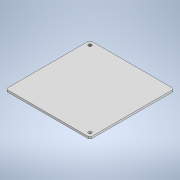
# Autodesk Inventor part: tampa caixa box
Saved by Autodesk Inventor 2022 (Build 260153000, 153)
## iProperties
Created: 2022-04-15
Part Number: tampa caixa box
Material: Genérico
Document SubType Name: Modeling
Designer: Hanter
Density: 1 g/cm^3
Appearance: Padrão
Author: Hanter
Autodesk Inventor part; units mm, degrees
ref_plane "YZ Plane" through (0, 0, 0) normal (1, 0, 0) x (0, 1, 0)
ref_plane "XZ Plane" through (0, 0, 0) normal (0, 1, 0) x (-1, 0, 0)
ref_plane "XY Plane" through (0, 0, 0) normal (0, 0, 1) x (1, 0, 0)
sketch "Esboço1" plane through (0, 0, 0) normal (0, 1, 0) x (-1, 0, 0)
  line L0 (-42.5, 42.5) -> (42.5, 42.5)
  line L1 (42.5, 42.5) -> (42.5, -42.5)
  line L2 (42.5, -42.5) -> (-42.5, -42.5)
  line L3 (-42.5, -42.5) -> (-42.5, 42.5)
  line L4 (-42.5, 42.5) -> (42.5, -42.5) construction
  line L5 (42.5, 42.5) -> (-42.5, -42.5) construction
  point P0 (0, 0)
  dimension "d0" = 85
  dimension "d1" = 85
  constraints: 12 end point, 2 midpoint, 2 parallel, 1 horizontal, 1 perpendicular
  measures "d0" distance of L1.end L2.end
  measures "d1" distance of L0.end L1.end
extrude "Extrusão1" add sketch "Esboço1" along normal blind 2
fillet "Arredondamento1" radius 2 4 edges at (42.5, 1, 42.5) (42.5, 1, -42.5) (-42.5, 1, 42.5) (-42.5, 1, -42.5)
sketch "Esboço2" plane through (0, 2, 0) normal (0, 1, 0) x (1, 0, 0)
  circle A0 centre (38.25, -38.25) radius 1.6
  line L0 (-40.5, -42.5) -> (40.5, -42.5) projected
  line L1 (42.5, -40.5) -> (42.5, 40.5) projected
  circle A1 centre (-38.25, 38.25) radius 1.6
  line L2 (-42.5, 40.5) -> (-42.5, -40.5) projected
  line L3 (40.5, 42.5) -> (-40.5, 42.5) projected
  point P0 (0, 0)
  dimension "d5" = 3.2
  dimension "d6" = 4.25
  dimension "d7" = 4.25
  dimension "d8" = 3.2
  dimension "d9" = 4.25
  dimension "d10" = 4.25
  constraints: 2 centre point
  measures "d5" diameter of A0
  measures "d6" distance from line of L0 A0.centre
  measures "d7" distance from line of L1 A0.centre
  measures "d8" diameter of A1
  measures "d9" distance from line of L2 A1.centre
  measures "d10" distance from line of L3 A1.centre
extrude "Extrusão2" cut sketch "Esboço2" against normal blind 2
